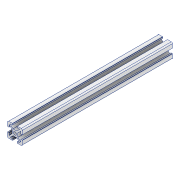
# Autodesk Inventor part: 2020 Aluminium Extrusion T-Slot lower arm
Saved by Autodesk Inventor 2021 (Build 250183000, 183)
## iProperties
Created: 2019-11-21
Part Number: 2020 Aluminium Extrusion T-Slot lower arm
Material: Aluminum 6061
Document SubType Name: Modeling
Designer: Johnson Ebenezer R
Density: 2.7 g/cm^3
Appearance: Aluminum - Flat
Author: Johnson Ebenezer R
Autodesk Inventor part; units mm, degrees
ref_plane "YZ Plane" through (0, 0, 0) normal (1, 0, 0) x (0, 1, 0)
ref_plane "XZ Plane" through (0, 0, 0) normal (0, 1, 0) x (-1, 0, 0)
ref_plane "XY Plane" through (0, 0, 0) normal (0, 0, 1) x (1, 0, 0)
sketch "Sketch1" plane through (0, 0, 0) normal (0, 0, 1) x (1, 0, 0)
  line L0 (-10, 10) -> (10, 10) construction
  line L1 (10, 10) -> (10, -10) construction
  line L2 (10, -10) -> (-10, -10) construction
  line L3 (-10, -10) -> (-10, 10) construction
  line L4 (-10, 10) -> (10, -10) construction
  line L5 (10, 10) -> (-10, -10) construction
  circle A0 centre (0, 0) radius 2
  line L6 (-4, -4) -> (4, -4) construction
  line L7 (4, -4) -> (4, 4) construction
  line L8 (4, 4) -> (-4, 4) construction
  line L9 (-4, 4) -> (-4, -4) construction
  line L10 (-4, -4) -> (4, 4) construction
  line L11 (4, -4) -> (-4, 4) construction
  line L12 (2.6444, 4.0586) -> (6.2444, 7.6586)
  line L13 (6.1029, 8) -> (3.3, 8)
  line L14 (3.1, 8.2) -> (3.1, 9.8)
  line L15 (3.3, 10) -> (8.5, 10)
  line L16 (4.0586, 2.6444) -> (7.6586, 6.2444)
  line L17 (8, 6.1029) -> (8, 3.3)
  line L18 (8.2, 3.1) -> (9.8, 3.1)
  line L19 (10, 8.5) -> (10, 3.3)
  line L20 (0, 4) -> (2.5029, 4)
  line L21 (4, 0) -> (4, 2.5029)
  line L22 (0, 10) -> (0, -10) construction
  line L23 (-10, 0) -> (10, 0) construction
  line L24 (-2.6444, 4.0586) -> (-6.2444, 7.6586)
  line L25 (-6.1029, 8) -> (-3.3, 8)
  line L26 (-3.1, 8.2) -> (-3.1, 9.8)
  line L27 (-3.3, 10) -> (-8.5, 10)
  line L28 (-4.0586, 2.6444) -> (-7.6586, 6.2444)
  line L29 (-8, 6.1029) -> (-8, 3.3)
  line L30 (-8.2, 3.1) -> (-9.8, 3.1)
  line L31 (-10, 8.5) -> (-10, 3.3)
  line L32 (0, 4) -> (-2.5029, 4)
  line L33 (-4, 0) -> (-4, 2.5029)
  line L34 (2.6444, -4.0586) -> (6.2444, -7.6586)
  line L35 (6.1029, -8) -> (3.3, -8)
  line L36 (3.1, -8.2) -> (3.1, -9.8)
  line L37 (3.3, -10) -> (8.5, -10)
  line L38 (4.0586, -2.6444) -> (7.6586, -6.2444)
  line L39 (8, -6.1029) -> (8, -3.3)
  line L40 (8.2, -3.1) -> (9.8, -3.1)
  line L41 (10, -8.5) -> (10, -3.3)
  line L42 (0, -4) -> (2.5029, -4)
  line L43 (4, 0) -> (4, -2.5029)
  line L44 (0, -4) -> (-2.5029, -4)
  line L45 (-2.6444, -4.0586) -> (-6.2444, -7.6586)
  line L46 (-6.1029, -8) -> (-3.3, -8)
  line L47 (-3.1, -8.2) -> (-3.1, -9.8)
  line L48 (-3.3, -10) -> (-8.5, -10)
  line L49 (-4.0586, -2.6444) -> (-7.6586, -6.2444)
  line L50 (-4, 0) -> (-4, -2.5029)
  line L51 (-8, -6.1029) -> (-8, -3.3)
  line L52 (-8.2, -3.1) -> (-9.8, -3.1)
  line L53 (-10, -8.5) -> (-10, -3.3)
  arc A1 (10, 8.5) -> (8.5, 10) centre (8.5, 8.5) ccw
  arc A2 (-8.5, 10) -> (-10, 8.5) centre (-8.5, 8.5) ccw
  arc A3 (-10, -8.5) -> (-8.5, -10) centre (-8.5, -8.5) ccw
  arc A4 (8.5, -10) -> (10, -8.5) centre (8.5, -8.5) ccw
  arc A5 (-3.1, 9.8) -> (-3.3, 10) centre (-3.3, 9.8) ccw
  arc A6 (-3.3, 8) -> (-3.1, 8.2) centre (-3.3, 8.2) ccw
  arc A7 (-6.1029, 8) -> (-6.2444, 7.6586) centre (-6.1029, 7.8) ccw
  arc A8 (6.2444, 7.6586) -> (6.1029, 8) centre (6.1029, 7.8) ccw
  arc A9 (-8, -6.1029) -> (-7.6586, -6.2444) centre (-7.8, -6.1029) ccw
  arc A10 (-3.1, -8.2) -> (-3.3, -8) centre (-3.3, -8.2) ccw
  arc A11 (6.1029, -8) -> (6.2444, -7.6586) centre (6.1029, -7.8) ccw
  arc A12 (3.3, -8) -> (3.1, -8.2) centre (3.3, -8.2) ccw
  arc A13 (-6.2444, -7.6586) -> (-6.1029, -8) centre (-6.1029, -7.8) ccw
  arc A14 (7.6586, -6.2444) -> (8, -6.1029) centre (7.8, -6.1029) ccw
  arc A15 (8.2, -3.1) -> (8, -3.3) centre (8.2, -3.3) ccw
  arc A16 (8, 6.1029) -> (7.6586, 6.2444) centre (7.8, 6.1029) ccw
  arc A17 (8, 3.3) -> (8.2, 3.1) centre (8.2, 3.3) ccw
  arc A18 (3.3, 10) -> (3.1, 9.8) centre (3.3, 9.8) ccw
  arc A19 (-2.6444, 4.0586) -> (-2.5029, 4) centre (-2.5029, 4.2) ccw
  arc A20 (2.5029, 4) -> (2.6444, 4.0586) centre (2.5029, 4.2) ccw
  arc A21 (4.0586, 2.6444) -> (4, 2.5029) centre (4.2, 2.5029) ccw
  arc A22 (4, -2.5029) -> (4.0586, -2.6444) centre (4.2, -2.5029) ccw
  arc A23 (2.6444, -4.0586) -> (2.5029, -4) centre (2.5029, -4.2) ccw
  arc A24 (-2.5029, -4) -> (-2.6444, -4.0586) centre (-2.5029, -4.2) ccw
  arc A25 (-4.0586, -2.6444) -> (-4, -2.5029) centre (-4.2, -2.5029) ccw
  arc A26 (-4, 2.5029) -> (-4.0586, 2.6444) centre (-4.2, 2.5029) ccw
  arc A27 (-7.6586, 6.2444) -> (-8, 6.1029) centre (-7.8, 6.1029) ccw
  arc A28 (-8.2, 3.1) -> (-8, 3.3) centre (-8.2, 3.3) ccw
  arc A29 (-10, 3.3) -> (-9.8, 3.1) centre (-9.8, 3.3) ccw
  arc A30 (-8, -3.3) -> (-8.2, -3.1) centre (-8.2, -3.3) ccw
  arc A31 (-9.8, -3.1) -> (-10, -3.3) centre (-9.8, -3.3) ccw
  arc A32 (-3.3, -10) -> (-3.1, -9.8) centre (-3.3, -9.8) ccw
  arc A33 (3.1, -9.8) -> (3.3, -10) centre (3.3, -9.8) ccw
  arc A34 (10, -3.3) -> (9.8, -3.1) centre (9.8, -3.3) ccw
  arc A35 (9.8, 3.1) -> (10, 3.3) centre (9.8, 3.3) ccw
  arc A36 (3.1, 8.2) -> (3.3, 8) centre (3.3, 8.2) ccw
  point P0 (2.5858, 4)
  point P1 (6.5858, 8)
  point P2 (3.1, 8)
  point P3 (3.1, 10)
  point P4 (4, 2.5858)
  point P5 (8, 6.5858)
  point P6 (8, 3.1)
  point P7 (10, 3.1)
  point P8 (-2.5858, 4)
  point P9 (-6.5858, 8)
  point P10 (-3.1, 8)
  point P11 (-3.1, 10)
  point P12 (-4, 2.5858)
  point P13 (-8, 6.5858)
  point P14 (-8, 3.1)
  point P15 (-10, 3.1)
  point P16 (2.5858, -4)
  point P17 (6.5858, -8)
  point P18 (3.1, -8)
  point P19 (3.1, -10)
  point P20 (4, -2.5858)
  point P21 (8, -6.5858)
  point P22 (8, -3.1)
  point P23 (10, -3.1)
  point P24 (-2.5858, -4)
  point P25 (-6.5858, -8)
  point P26 (-3.1, -8)
  point P27 (-3.1, -10)
  point P28 (-4, -2.5858)
  point P29 (-8, -6.5858)
  point P30 (-8, -3.1)
  point P31 (-10, -3.1)
  dimension "d0" = 20
  dimension "d1" = 20
  dimension "d2" = 4
  dimension "d5" = 6
  dimension "t" = 2
  dimension "d7" = 1
  dimension "d8" = 2
  dimension "d9" = 2
  dimension "d10" = 3.1
  dimension "d11" = 3.1
  dimension "d15" = 1.5
  dimension "d16" = 1.5
  dimension "d17" = 1.5
  dimension "d18" = 1.5
  dimension "d19" = 0.2
  dimension "d20" = 0.2
  dimension "d21" = 0.2
  dimension "d22" = 0.2
  dimension "d23" = 0.2
  dimension "d24" = 0.2
  dimension "d25" = 0.2
  dimension "d26" = 0.2
  dimension "d27" = 0.2
  dimension "d28" = 0.2
  dimension "d29" = 0.2
  dimension "d30" = 0.2
  dimension "d31" = 0.2
  dimension "d32" = 0.2
  dimension "d33" = 0.2
  dimension "d34" = 0.2
  dimension "d35" = 0.2
  dimension "d36" = 0.2
  dimension "d37" = 0.2
  dimension "d38" = 0.2
  dimension "d39" = 0.2
  dimension "d40" = 0.2
  dimension "d41" = 0.2
  constraints: 108 end point, 76 point on line, 72 point on circle, 72 tangent, 37 centre point, 26 symmetric about line, 10 midpoint, 9 equal radius, 6 parallel, 5 perpendicular, 3 horizontal, 2 collinear, 1 coincident, 1 vertical
  measures "d0" distance of L0.start L0.end
  measures "d1" distance of L0.end L1.end
  measures "d2" diameter of A0
  measures "d5" distance between parallel lines of L8 L0
  measures "t" distance between parallel lines of L12 L16
  measures "d7" distance between parallel lines of L12 L5
  measures "d8" distance between parallel lines of L13 L15
  measures "d9" distance between parallel lines of L19 L17
  measures "d10" distance from line of L14 L20.start
  measures "d11" distance from line of L18 L21.start
  measures "d15" radius of A1
  measures "d16" radius of A2
  measures "d17" radius of A3
  measures "d18" radius of A4
  measures "d19" radius of A5
  measures "d20" radius of A6
  measures "d21" radius of A7
  measures "d22" radius of A14
  measures "d23" radius of A16
  measures "d24" radius of A18
  measures "d25" radius of A19
  measures "d26" radius of A20
  measures "d27" radius of A21
  measures "d28" radius of A22
  measures "d29" radius of A23
  measures "d30" radius of A24
  measures "d31" radius of A25
  measures "d32" radius of A26
  measures "d33" radius of A27
  measures "d34" radius of A28
  measures "d35" radius of A29
  measures "d36" radius of A31
  measures "d37" radius of A32
  measures "d38" radius of A33
  measures "d39" radius of A34
  measures "d40" radius of A35
  measures "d41" radius of A36
extrude "2020 Al T-S (1000mm)" add sketch "Sketch1" along normal blind 203.2
equation "\"d1\" = d0"
equation "\"d7\" = 0.5 * t"
equation "\"d8\" = t"
equation "\"d9\" = t"
equation "\"d11\" = d10"
body "Solid1"
